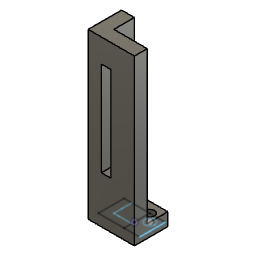
limitswitchflagholder (Autodesk Fusion 360 design; units mm, degrees)
Autodesk Fusion 360 part; units mm, degrees
note: some values were not read from the file. Set by a fixed rule: which sketch regions a step uses.
sketch "Sketch1" plane through (0, 0, 0) normal (0, 1, 0) x (1, 0, 0)
  line L0 (6, 0) -> (6, 6)
  line L1 (6, 6) -> (0, 6)
  line L2 (0, 6) -> (0, 0)
  circle A0 centre (3, 3) radius 1.85
  line L3 (0, 0) -> (0, -4)
  line L4 (6, 0) -> (6, -4)
  line L5 (6, -4) -> (0, -4)
  line L6 (0, -4) -> (-10, -4)
  line L7 (-10, -4) -> (-10, 6)
  line L8 (-10, 6) -> (0, 6)
  line L9 (-5, -1) -> (0, -1)
  line L10 (-7, 2.1291) -> (-7, 6)
  line L11 (-5, -1) -> (-7, -1)
  line L12 (-7, 2.1291) -> (-7, -1)
  dimension "d4" = 6
  dimension "d5" = 6
  dimension "d6" = 3.7
  dimension "d8" = 4
  dimension "d10" = 10
  dimension "d11" = 10
  constraint vertical L0
  constraint horizontal L1
  constraint vertical L2
  constraint coincident L2.end L3.start
  constraint parallel L2 L3
  constraint parallel L3 L4
  constraint perpendicular L3 L5
  constraint perpendicular L3 L6
  constraint perpendicular L6 L7
  constraint coincident L3 L9.end
  constraint perpendicular L3 L9
  constraint coincident L8 L10.end
  constraint perpendicular L8 L10
  constraint perpendicular L11 L12
  measures "d4" distance of L2.end L0.start
  measures "d5" distance of L2.end L1.end
  measures "d6" diameter of A0
  measures "d8" distance of L2.end L3.end
  measures "d10" distance of L3.end L6.end
  measures "d11" distance of L6.end L7.end
extrude "Extrude2" add sketch "Sketch1" along normal blind 3 contours L0 L1 L2 L3 L4 L5 | L2 L3 L8 L9 L10 L11 L12 makes body 1
extrude "Extrude1" add sketch "Sketch1" along normal blind 62 separate body contours L3 L6 L7 L8 L9 L10 L11 L12 makes body 2
sketch "Sketch2" plane through (-10, 0, 0) normal (-1, 0, 0) x (0, 0, 1)
  line L0 (-6, 0) -> (4, 0)
  line L1 (4, 0) -> (4, 62)
  line L2 (4, 62) -> (-6, 62)
  line L3 (-6, 62) -> (-6, 0)
  circle A0 centre (-1, 57.5) radius 1.85
  line L4 (-1, 0) -> (-1, 4.5)
  circle A1 centre (-1, 4.5) radius 1.85
  line L5 (-2.85, 4.5) -> (-2.85, 57.5)
  line L6 (0.85, 57.5) -> (0.85, 4.5)
  dimension "d21" = 3.7
  dimension "d22" = 4.5
  dimension "d23" = 3.7
  constraint midpoint L0 L4.start
  constraint perpendicular L0 L4
  constraint coincident L4.end A1.centre
  constraint coincident A1 L5.start
  constraint coincident A0 L5.end
  constraint tangent A0 L5
  constraint parallel L4 L5
  constraint coincident A0 L6.start
  constraint coincident A1 L6.end
  constraint tangent A1 L6
  constraint perpendicular L0 L6
  measures "d21" diameter of A0
  measures "d22" distance of L4.start L4.end
  measures "d23" diameter of A1
extrude "Extrude3" cut sketch "Sketch2" against normal up to surface (3 mm away) contours A0 | A0 A1 L5 L6 | A1 bodies 2
sketch "Sketch3" plane through (0, 0, 4) normal (0, 0, 1) x (1, 0, 0)
  line L0 (-10, 0) -> (0, 0)
  line L1 (0, 0) -> (0, 62)
  line L2 (0, 62) -> (-10, 62)
  line L3 (-10, 62) -> (-10, 0)
  line L4 (-5, 62) -> (-5, 57.5)
  line L5 (-5, 0) -> (-5, 4.5)
  line L6 (-3.15, 57.5) -> (-3.15, 4.5)
  line L7 (-6.85, 57.5) -> (-6.85, 4.5)
  line L8 (-6.85, 52.8937) -> (-3.15, 52.8937)
  line L9 (-6.85, 16.2389) -> (-3.15, 16.2389)
  dimension "d26" = 4.5
  dimension "d28" = 4.5
  constraint midpoint L2 L4.start
  constraint perpendicular L2 L4
  constraint midpoint L0 L5.start
  constraint perpendicular L0 L5
  constraint perpendicular L0 L6
  constraint perpendicular L0 L7
  constraint coincident L7 L8.start
  constraint coincident L6 L8.end
  constraint perpendicular L6 L8
  constraint coincident L7 L9.start
  constraint coincident L6 L9.end
  constraint perpendicular L6 L9
  measures "d26" distance of L4.start L4.end
  measures "d28" distance of L5.start L5.end
extrude "Extrude4" cut sketch "Sketch3" against normal up to surface (3 mm away) contours L6 L7 L8 L9 bodies 2
sketch "Sketch4" plane through (0, 0, -6) normal (0, 0, -1) x (-1, 0, 0)
  line L0 (7, 0) -> (10, 0)
  line L1 (10, 0) -> (10, 62)
  line L2 (10, 62) -> (7, 62)
  line L3 (7, 62) -> (7, 0)
sketch "Sketch5" plane through (0, 0, 0) normal (0, 1, 0) x (1, 0, 0)
extrude "Extrude5" add sketch "Sketch1" against normal blind 2 bodies 1 2
sketch "Sketch6" plane through (-10, 0, 0) normal (-1, 0, 0) x (0, 0, 1)
  line L0 (-2.85, 4.5) -> (-2.85, 57.5)
  arc A0 (0.85, 57.5) -> (-2.85, 57.5) centre (-1, 57.5) ccw
  line L1 (0.85, 57.5) -> (0.85, 4.5)
  arc A1 (-2.85, 4.5) -> (0.85, 4.5) centre (-1, 4.5) ccw
  line L2 (4, -2) -> (4, 62)
  line L3 (4, 62) -> (-6, 62)
  line L4 (-6, 62) -> (-6, -2)
  line L5 (-6, -2) -> (4, -2)
  line L6 (-2.85, 49.1228) -> (0.85, 49.1228)
  line L7 (-2.85, 15.8582) -> (0.85, 15.8582)
  constraint coincident L0 L6.start
  constraint coincident L1 L6.end
  constraint perpendicular L1 L6
  constraint coincident L0 L7.start
  constraint coincident L1 L7.end
  constraint perpendicular L1 L7
extrude "Extrude6" add sketch "Sketch6" against normal up to surface (3 mm away) contours L0 L1 A1 L7 | L0 A0 L1 L6 bodies 1
extrude "Extrude7" add 1 faces at (0, 22.6667, 2) along direction (1, 0, 0) up to surface (6 mm away) on bodies 1 bodies 1
extrude "Extrude8" add sketch "Sketch4" 1 faces at (-3.6667, -0.3333, -6) along normal blind 1 on bodies 1 bodies 1
move_face "OffsetFaces1" offset 2 2 faces at (-10, 3.9527, -1.95) (-2.3833, 4.0796, 4) on bodies 1
